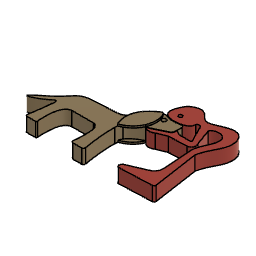
Dog+Human v3 (Autodesk Fusion 360 design; units mm, degrees)
Autodesk Fusion 360 part; units mm, degrees
sketch "Sketch2" plane through (0, 0, 0) normal (0, 0, 1) x (1, 0, 0)
  line L0 (48.3178, -14.7986) -> (66.8883, -14.0451)
  arc A0 (48, -12) -> (47.2858, -13.6689) centre (50.6178, -14.1075) ccw
  line L1 (48, -12) -> (58.7244, -7.4038)
  line L2 (61.7417, -2.4457) -> (60.5774, 13.5743)
  arc A1 (58.7244, -7.4038) -> (61.7417, -2.4457) centre (56.7548, -2.8081) ccw
  line L3 (67.8369, -12.8994) -> (64, 13)
  arc A2 (66.8883, -14.0451) -> (67.8369, -12.8994) centre (66.8477, -13.0459) ccw
  arc A3 (47.2858, -13.6689) -> (48.3178, -14.7986) centre (48.2773, -13.7994) ccw
  spline S0 degree 5 poles (64, 13) (64.0471, 13.236) (64.1458, 13.7046) (64.307, 14.397) (64.5486, 15.2992) (64.8941, 16.3923) (65.2816, 17.4521) (65.7073, 18.4807) (66.1652, 19.4823) (66.6461, 20.4629) (67.1375, 21.4305) (67.6248, 22.3939) (68.0914, 23.3623) (68.5198, 24.344) (68.8918, 25.3461) (69.1895, 26.3733) (69.3965, 27.4267) (69.4986, 28.5028) (69.4851, 29.5927) (69.3499, 30.6803) (69.0922, 31.7424) (68.7145, 32.7515) (68.2224, 33.6784) (67.6229, 34.495) (66.923, 35.1766) (66.1295, 35.7045) (65.2494, 36.0668) (64.2908, 36.2591) (63.2636, 36.2857) (62.18, 36.1608) (61.055, 35.9071) (59.905, 35.5526) (58.7478, 35.1288) (57.6019, 34.6678) (56.4863, 34.1999) (55.4192, 33.7519) (54.4162, 33.3481) (53.4883, 33.0109) (52.6395, 32.7617) (51.8652, 32.6219) (51.15, 32.613) (50.4738, 32.7518) (49.816, 33.047) (49.1613, 33.4942) (48.4996, 34.0735) (47.8215, 34.7497) (47.1154, 35.4716) (46.362, 36.1698) (45.5357, 36.7621) (44.6155, 37.1708) (43.5952, 37.3392) (42.4916, 37.2453) (41.3588, 36.9242) (40.2766, 36.4544) (39.3246, 35.924) (38.5591, 35.4018) (37.9922, 34.91) (37.5608, 34.3854) (37.1497, 33.7029) (36.6699, 32.7597) (36.0857, 31.5062) (35.5413, 30.0769) (35.2161, 28.6525) (35.1938, 27.3301) (35.5233, 26.1827) (36.205, 25.246) (37.2092, 24.5352) (38.4805, 24.0502) (39.9471, 23.7826) (41.5263, 23.7169) (43.1305, 23.8338) (44.6732, 24.1116) (46.0752, 24.5292) (47.2705, 25.0683) (48.2132, 25.7157) (48.8766, 26.4637) (49.1732, 27.1395) (49.262, 27.6892) (49.2618, 28.0748) (49.2469, 28.2723) knots 0 0 0 0 0 0 0.01333333 0.02666667 0.04 0.05333333 0.06666667 0.08 0.09333333 0.10666667 0.12 0.13333333 0.14666667 0.16 0.17333333 0.18666667 0.2 0.21333333 0.22666667 0.24 0.25333333 0.26666667 0.28 0.29333333 0.30666667 0.32 0.33333333 0.34666667 0.36 0.37333333 0.38666667 0.4 0.41333333 0.42666667 0.44 0.45333333 0.46666667 0.48 0.49333333 0.50666667 0.52 0.53333333 0.54666667 0.56 0.57333333 0.58666667 0.6 0.61333333 0.62666667 0.64 0.65333333 0.66666667 0.68 0.69333333 0.70666667 0.72 0.73333333 0.74666667 0.76 0.77333333 0.78666667 0.8 0.81333333 0.82666667 0.84 0.85333333 0.86666667 0.88 0.89333333 0.90666667 0.92 0.93333333 0.94666667 0.96 0.97333333 0.98666667 1 1 1 1 1 1
  arc A4 (51.7725, 28.2723) -> (49.2469, 28.2723) centre (50.5097, 27.6397) ccw
  line L4 (51.7725, 28.2723) -> (56.2933, 19.2488)
  line L5 (55.8463, 18.5249) -> (49.7974, 18.5249)
  arc A5 (55.8463, 18.5249) -> (56.2933, 19.2488) centre (55.8463, 19.0249) ccw
  arc A6 (36.5352, 12.6034) -> (41.8633, 12.6034) centre (39.1992, 15.9969) ccw
  line L6 (36.5352, 12.6034) -> (45.5261, 16.9194)
  arc A7 (45.5261, 16.9194) -> (47.0032, 19.5393) centre (44.3899, 19.2864) ccw
  line L7 (49.2932, 18.6613) -> (47.3781, 19.7793)
  arc A8 (49.2932, 18.6613) -> (49.7974, 18.5249) centre (49.7974, 19.5249) ccw
  arc A9 (47.3781, 19.7793) -> (47.0032, 19.5393) centre (47.2521, 19.5634) ccw
  line L8 (41.8633, 12.6034) -> (47.1907, 14.7614)
  line L9 (47.1907, 14.7614) -> (57.3572, 15.166)
  arc A10 (57.3572, 15.166) -> (59.3412, 19.3874) centre (57.2527, 17.7921) ccw
  line L10 (55.9993, 28.5525) -> (59.3412, 19.3874)
  spline S1 degree 5 poles (55.9993, 28.5525) (56.0014, 28.6403) (56.0224, 28.8148) (56.1046, 29.0731) (56.3157, 29.4108) (56.7472, 29.8172) (57.3391, 30.1944) (58.0744, 30.5148) (58.9263, 30.7421) (59.8582, 30.8379) (60.8246, 30.768) (61.7699, 30.5098) (62.6312, 30.0565) (63.3465, 29.4128) (63.8634, 28.5934) (64.1466, 27.6199) (64.1876, 26.5191) (64.0077, 25.3203) (63.6477, 24.0543) (63.1622, 22.7518) (62.6114, 21.4416) (62.0548, 20.1495) (61.5441, 18.8963) (61.1155, 17.6964) (60.7919, 16.559) (60.5861, 15.4889) (60.5203, 14.6883) (60.5271, 14.1191) (60.5565, 13.7536) (60.5774, 13.5743) knots 0 0 0 0 0 0 0.04 0.08 0.12 0.16 0.2 0.24 0.28 0.32 0.36 0.4 0.44 0.48 0.52 0.56 0.6 0.64 0.68 0.72 0.76 0.8 0.84 0.88 0.92 0.96 1 1 1 1 1 1
  line L11 (36.6253, 12.924) -> (45.4179, 17.1448)
  arc A11 (45.4179, 17.1448) -> (46.7544, 19.5152) centre (44.3899, 19.2864) ccw
  line L12 (46.7544, 19.5152) -> (46.7544, 23)
  spline S2 degree 3 poles (38.1614, 23.9293) (38.1637, 23.9282) (38.166, 23.927) (38.1682, 23.9259) (38.8344, 23.59) (39.8483, 23.4934) (41.1161, 23.5073) (42.4706, 23.5221) (44.0665, 23.6811) (45.4723, 24.0408) knots 0.849842 0.849842 0.849842 0.849842 0.84997 0.84997 0.84997 0.887416 0.887416 0.887416 0.92742 0.92742 0.92742 0.92742
  spline S3 degree 5 poles (38.1614, 23.9293) (38.0904, 23.9626) (37.9463, 24.0275) (37.7243, 24.1199) (37.4165, 24.2331) (37.012, 24.3571) (36.5877, 24.4612) (36.1436, 24.5414) (35.6807, 24.5905) (35.2003, 24.5996) (34.7049, 24.5597) (34.1981, 24.4629) (33.685, 24.3041) (33.1725, 24.083) (32.6687, 23.8027) (32.1817, 23.4686) (31.7196, 23.087) (31.2889, 22.6644) (30.8942, 22.206) (30.5378, 21.7155) (30.2209, 21.1956) (29.999, 20.7573) (29.8502, 20.4163) (29.7589, 20.1836) (29.7151, 20.0659) knots 0 0 0 0 0 0 0.05 0.1 0.15 0.2 0.25 0.3 0.35 0.4 0.45 0.5 0.55 0.6 0.65 0.7 0.75 0.8 0.85 0.9 0.95 1 1 1 1 1 1
  arc A12 (46.7544, 23) -> (45.4723, 24.0408) centre (45.6909, 23) ccw
  line L13 (36.2228, 12.9106) -> (36, 13)
  arc A13 (27.6529, 5.3934) -> (36, 13) centre (23.3259, 18.5248) ccw
  arc A14 (36.2228, 12.9106) -> (36.6253, 12.924) centre (36.4089, 13.3747) ccw
  circle A15 centre (40.6607, 28.1735) radius 1.021
  spline S4 degree 5 poles (27.6042, 3.833) (27.602, 3.6993) (27.5972, 3.3329) (27.594, 2.7215) (27.6001, 1.8426) (27.6274, 0.6635) (27.6817, -0.6876) (27.7608, -2.0969) (27.8648, -3.554) (27.9935, -5.0466) (28.1465, -6.5622) (28.3233, -8.0892) (28.5231, -9.6191) (28.7449, -11.1464) (28.9494, -12.4296) (29.1158, -13.4049) (29.2353, -14.0751) (29.3023, -14.4425) (29.3142, -14.5078) knots 0.094478 0.094478 0.094478 0.094478 0.094478 0.094478 0.133333 0.2 0.266667 0.333333 0.4 0.466667 0.533333 0.6 0.666667 0.733333 0.8 0.866667 0.933333 0.947774 0.947774 0.947774 0.947774 0.947774 0.947774
  spline S5 degree 5 poles (29.7151, 20.0659) (29.7034, 19.9832) (29.6746, 19.8136) (29.6152, 19.5469) (29.5031, 19.166) (29.3072, 18.6479) (29.0541, 18.0893) (28.7433, 17.4946) (28.3758, 16.8732) (27.9541, 16.2381) (27.4813, 15.6035) (26.9607, 14.9833) (26.3957, 14.3898) (25.7897, 13.8308) (25.1457, 13.3105) (24.4663, 12.8304) (23.896, 12.4785) (23.4536, 12.2324) (23.1523, 12.0761) (23, 12) knots 0 0 0 0 0 0 0.066667 0.133333 0.2 0.266667 0.333333 0.4 0.466667 0.533333 0.6 0.666667 0.733333 0.8 0.866667 0.933333 1 1 1 1 1 1
  line L14 (28.3306, -15.688) -> (23.2583, -15.688)
  arc A16 (28.3306, -15.688) -> (29.3142, -14.5078) centre (28.3306, -14.688) ccw
  spline S6 degree 5 poles (22.2762, -14.4996) (22.2937, -14.4079) (22.3426, -14.1433) (22.4165, -13.6959) (22.5039, -13.0476) (22.5884, -12.1739) (22.6483, -11.1641) (22.6776, -10.1178) (22.6815, -9.0523) (22.6668, -7.9917) (22.6403, -6.962) (22.607, -5.9886) (22.5685, -5.0925) (22.5211, -4.2869) (22.4537, -3.5727) (22.3483, -2.9392) (22.1852, -2.3699) (21.9451, -1.8467) (21.6139, -1.3544) (21.2642, -0.9715) (20.9529, -0.691) (20.7213, -0.5052) (20.5955, -0.41) (20.5869, -0.4035) knots 0.073114 0.073114 0.073114 0.073114 0.073114 0.073114 0.1 0.15 0.2 0.25 0.3 0.35 0.4 0.45 0.5 0.55 0.6 0.65 0.7 0.75 0.8 0.85 0.9 0.95 0.953696 0.953696 0.953696 0.953696 0.953696 0.953696
  arc A17 (22.2762, -14.4996) -> (23.2583, -15.688) centre (23.2583, -14.688) ccw
  spline S7 degree 5 poles (23, 12) (22.8644, 11.9727) (22.5949, 11.9202) (22.1952, 11.8479) (21.6715, 11.7643) (21.0295, 11.6804) (20.3913, 11.6155) (19.7391, 11.566) (19.0443, 11.5261) (18.2763, 11.4892) (17.4102, 11.4493) (16.434, 11.4022) (15.3575, 11.3469) (14.2059, 11.2848) (13.0146, 11.2184) (11.822, 11.1509) (10.6644, 11.0845) (9.5691, 11.0198) (8.5482, 10.9547) (7.6011, 10.8845) (6.7187, 10.802) (5.8886, 10.6979) (5.0981, 10.5613) (4.3399, 10.3791) (3.6122, 10.1382) (2.915, 9.8269) (2.2486, 9.4369) (1.6106, 8.9656) (0.9945, 8.4172) (0.3904, 7.8002) (-0.2137, 7.1253) (-0.8314, 6.4042) (-1.4768, 5.6467) (-2.1635, 4.8605) (-2.9029, 4.0519) (-3.7026, 3.2268) (-4.5649, 2.3911) (-5.485, 1.5515) (-6.4493, 0.7165) (-7.4359, -0.1039) (-8.4176, -0.8991) (-9.3652, -1.6583) (-10.2493, -2.3712) (-11.0438, -3.0293) (-11.7284, -3.6258) (-12.2912, -4.1568) (-12.6393, -4.5279) (-12.8423, -4.7758) (-12.9517, -4.9275) (-13, -5) knots 0 0 0 0 0 0 0.022222 0.044444 0.066667 0.088889 0.111111 0.133333 0.155556 0.177778 0.2 0.222222 0.244444 0.266667 0.288889 0.311111 0.333333 0.355556 0.377778 0.4 0.422222 0.444444 0.466667 0.488889 0.511111 0.533333 0.555556 0.577778 0.6 0.622222 0.644444 0.666667 0.688889 0.711111 0.733333 0.755556 0.777778 0.8 0.822222 0.844444 0.866667 0.888889 0.911111 0.933333 0.955556 0.977778 1 1 1 1 1 1
  line L15 (19.3823, 0) -> (7, 0)
  arc A18 (20.5869, -0.4035) -> (19.3823, 0) centre (19.3823, -2) ccw
  spline S8 degree 5 poles (7, 0) (6.9194, -0.0106) (6.7585, -0.036) (6.5184, -0.0869) (6.2009, -0.1804) (5.8085, -0.3411) (5.4216, -0.5488) (5.0422, -0.809) (4.6736, -1.1304) (4.3195, -1.5224) (3.9844, -1.994) (3.6728, -2.5517) (3.389, -3.1985) (3.1369, -3.9332) (2.9197, -4.7508) (2.7395, -5.6427) (2.5971, -6.5958) (2.4917, -7.593) (2.4203, -8.6127) (2.3785, -9.6303) (2.361, -10.62) (2.362, -11.556) (2.3757, -12.4145) (2.3971, -13.1753) (2.422, -13.8233) (2.4482, -14.3503) (2.4691, -14.6725) (2.4846, -14.858) (2.4949, -14.9568) (2.5, -15) knots 0 0 0 0 0 0 0.04 0.08 0.12 0.16 0.2 0.24 0.28 0.32 0.36 0.4 0.44 0.48 0.52 0.56 0.6 0.64 0.68 0.72 0.76 0.8 0.84 0.88 0.92 0.96 1 1 1 1 1 1
  line L16 (2.1088, -15.688) -> (-3, -15.688)
  arc A19 (2.1088, -15.688) -> (2.5, -15) centre (2.1088, -15.2328) ccw
  spline S9 degree 5 poles (-13, -5) (-13.0435, -5.0603) (-13.1155, -5.1721) (-13.1785, -5.313) (-13.1726, -5.4473) (-13.016, -5.5258) (-12.714, -5.5149) (-12.2753, -5.4157) (-11.713, -5.2303) (-11.0438, -4.9629) (-10.2882, -4.6193) (-9.4694, -4.2083) (-8.6131, -3.7416) (-7.7476, -3.2342) (-6.9029, -2.7056) (-6.1081, -2.1769) (-5.3897, -1.6695) (-4.7688, -1.2034) (-4.259, -0.7949) (-3.8636, -0.4553) (-3.5735, -0.1887) (-3.3642, 0.0098) (-3.1943, 0.1557) (-3.0212, 0.2651) (-2.814, 0.3473) (-2.5716, 0.3929) (-2.3181, 0.3778) (-2.088, 0.2729) (-1.9127, 0.0531) (-1.8116, -0.297) (-1.7961, -0.786) (-1.8564, -1.2913) (-1.9431, -1.7347) (-2.0193, -2.0589) (-2.062, -2.2282) knots 0 0 0 0 0 0 0.033333 0.066667 0.1 0.133333 0.166667 0.2 0.233333 0.266667 0.3 0.333333 0.366667 0.4 0.433333 0.466667 0.5 0.533333 0.566667 0.6 0.633333 0.666667 0.7 0.733333 0.766667 0.8 0.833333 0.866667 0.9 0.933333 0.966667 1 1 1 1 1 1
  spline S10 degree 5 poles (-2.062, -2.2282) (-2.0691, -2.3905) (-2.085, -2.7172) (-2.1137, -3.2132) (-2.1621, -3.8867) (-2.2396, -4.749) (-2.3339, -5.6311) (-2.4442, -6.531) (-2.5685, -7.4447) (-2.7031, -8.3651) (-2.843, -9.2835) (-2.9831, -10.1903) (-3.1183, -11.0766) (-3.2443, -11.9348) (-3.3586, -12.7606) (-3.4599, -13.5523) (-3.5303, -14.1582) (-3.5772, -14.5974) (-3.6058, -14.8835) (-3.6194, -15.0248) knots 0 0 0 0 0 0 0.066667 0.133333 0.2 0.266667 0.333333 0.4 0.466667 0.533333 0.6 0.666667 0.733333 0.8 0.866667 0.933333 1 1 1 1 1 1
  arc A20 (-3.6194, -15.0248) -> (-3, -15.688) centre (-3, -15.0671) ccw
  circle A21 centre (38.0321, 21.4887) radius 1.2353
  spline S11 degree 5 poles (28.657, 7.4803) (28.6665, 7.4959) (28.7314, 7.6021) (28.8531, 7.7936) (29.0355, 8.0595) (29.2866, 8.386) (29.6135, 8.755) (29.9756, 9.1162) (30.3812, 9.4834) (30.8349, 9.8666) (31.3354, 10.2687) (31.874, 10.6838) (32.4378, 11.1005) (33.0115, 11.5043) (33.5797, 11.88) (34.1289, 12.2141) (34.6499, 12.4978) (35.1381, 12.7265) (35.5005, 12.8642) (35.7564, 12.942) (35.92, 12.9825) (36, 13) knots 0.191487 0.191487 0.191487 0.191487 0.191487 0.191487 0.2 0.25 0.3 0.35 0.4 0.45 0.5 0.55 0.6 0.65 0.7 0.75 0.8 0.85 0.9 0.95 1 1 1 1 1 1
  arc A22 (28.657, 7.4803) -> (27.6042, 3.833) centre (34.8532, 3.7161) ccw
  spline S12 degree 5 poles (27.6529, 5.3934) (27.5917, 5.5238) (27.4722, 5.787) (27.3016, 6.1893) (27.0915, 6.7405) (26.8583, 7.4542) (26.6562, 8.1925) (26.4881, 8.9545) (26.3586, 9.7387) (26.2744, 10.5428) (26.2431, 11.3628) (26.2709, 12.1929) (26.361, 13.0245) (26.512, 13.8461) (26.7157, 14.6418) (26.9575, 15.3934) (27.2217, 16.0842) (27.495, 16.7037) (27.7703, 17.2505) (28.0523, 17.7383) (28.3566, 18.1947) (28.7027, 18.6509) (29.1081, 19.1349) (29.5815, 19.6613) (30.1188, 20.2273) (30.7077, 20.8181) (31.3311, 21.4121) (31.9707, 21.9853) (32.61, 22.5162) (33.2379, 22.9909) (33.8482, 23.4014) (34.3198, 23.6753) (34.6637, 23.8497) (34.8886, 23.9522) (35, 24) knots 0 0 0 0 0 0 0.033333 0.066667 0.1 0.133333 0.166667 0.2 0.233333 0.266667 0.3 0.333333 0.366667 0.4 0.433333 0.466667 0.5 0.533333 0.566667 0.6 0.633333 0.666667 0.7 0.733333 0.766667 0.8 0.833333 0.866667 0.9 0.933333 0.966667 1 1 1 1 1 1
  spline S13 degree 5 poles (36, 13) (36.0341, 13.0718) (36.1014, 13.2206) (36.1999, 13.4596) (36.3265, 13.8101) (36.4763, 14.3014) (36.6161, 14.8448) (36.7436, 15.4377) (36.8547, 16.0741) (36.9438, 16.7448) (37.0046, 17.4388) (37.0314, 18.1437) (37.0191, 18.8471) (36.9647, 19.5371) (36.8684, 20.2038) (36.7326, 20.8385) (36.5612, 21.4347) (36.3588, 21.9871) (36.13, 22.4919) (35.8784, 22.9471) (35.6062, 23.3521) (35.373, 23.636) (35.1897, 23.8267) (35.0639, 23.9439) (35, 24) knots 0 0 0 0 0 0 0.05 0.1 0.15 0.2 0.25 0.3 0.35 0.4 0.45 0.5 0.55 0.6 0.65 0.7 0.75 0.8 0.85 0.9 0.95 1 1 1 1 1 1
  line L17 (38.6901, 37.6299) -> (33.5795, 25.4813)
  point P0 (65.9185, 18.9318)
  point P1 (68.3564, 23.9877)
  point P2 (69.4704, 29.3006)
  point P3 (67.7566, 34.2708)
  point P4 (64, 36.2418)
  point P5 (57.9019, 34.785)
  point P6 (52.7603, 32.814)
  point P7 (50.1895, 32.8997)
  point P8 (47.3616, 35.2134)
  point P9 (43.1627, 37.2701)
  point P10 (38.3639, 35.2134)
  point P11 (36.1348, 31.5556)
  point P12 (36.8398, 24.8521)
  point P13 (46.4504, 24.7283)
  point P14 (56.8626, 29.8657)
  point P15 (60.5293, 30.7628)
  point P16 (64, 28)
  point P17 (62, 20)
  point P18 (36.4369, 24.4844)
  point P19 (34.1571, 24.4374)
  point P20 (31.5483, 22.9097)
  point P21 (27.6529, 0.1014)
  point P22 (28.2549, -7.4728)
  point P23 (29, 18)
  point P24 (26.74, 14.7614)
  point P25 (22.6616, -10.5608)
  point P26 (22.5451, -4.7345)
  point P27 (22, -2)
  point P28 (20.5071, 11.6302)
  point P29 (17.3179, 11.4444)
  point P30 (10.475, 11.0729)
  point P31 (5.5827, 10.6394)
  point P32 (2.4244, 9.5247)
  point P33 (-0.5171, 6.7689)
  point P34 (-5, 2)
  point P35 (-11, -3)
  point P36 (5.5276, -0.5003)
  point P37 (4, -2)
  point P38 (2.6007, -6.6518)
  point P39 (2.398, -13.1474)
  point P40 (-13, -5.5)
  point P41 (-8.7069, -3.7856)
  point P42 (-3.6194, -0.2295)
  point P43 (-2.9445, 0.2896)
  point P44 (-2.1658, 0.2896)
  point P45 (-2.4514, -6.5629)
  point P46 (-3.1522, -11.313)
  point P47 (29, 8)
  point P48 (30.7092, 9.7573)
  point P49 (33.7462, 11.9769)
  point P50 (26.4858, 9.0233)
  point P51 (26.4476, 13.4549)
  point P52 (27.6529, 17.0078)
  point P53 (29, 19)
  point P54 (32, 22)
  point P55 (36.6856, 15.1825)
  point P56 (37, 19)
  point P57 (36.2228, 22.2741)
  dimension "d1" = 5
  dimension "d2" = 1
  dimension "d3" = 0.5
  dimension "d4" = 1
  dimension "d5" = 0.25
  dimension "d8" = 0.5
  dimension "d11" = 1
  dimension "d12" = 1
  dimension "d13" = 2
  dimension "d14" = 7.25
  constraint tangent L1 A1
  constraint tangent L2 A1
  constraint tangent L0 A2
  constraint tangent L3 A2
  constraint tangent L0 A3
  constraint tangent A0 A3
  constraint equal A2 A3
  constraint tangent A4 L4
  constraint horizontal L5
  constraint tangent L4 A5
  constraint tangent L5 A5
  constraint tangent L6 A7
  constraint tangent L5 A8
  constraint tangent L7 A8
  constraint tangent A7 A9
  constraint tangent L7 A9
  constraint tangent L9 A10
  constraint vertical L12
  constraint tangent L12 A12
  constraint concentric A7 A11
  constraint tangent L11 A11
  constraint tangent L11 A14
  constraint tangent L13 A14
  constraint horizontal L14
  constraint tangent S4 A16
  constraint tangent L14 A16
  constraint tangent L14 A17
  constraint tangent S6 A17
  constraint horizontal L15
  constraint tangent S6 A18
  constraint tangent L15 A18
  constraint parallel L14 L16
  constraint tangent L16 A19
  constraint tangent L16 A20
  constraint tangent S11 A22
  constraint tangent S4 A22
  constraint midpoint P11 L17
  measures "d1" radius of A1
  measures "d2" radius of A2
  measures "d3" radius of A5
  measures "d4" radius of A8
  measures "d5" radius of A9
  measures "d8" radius of A14
  measures "d11" radius of A16
  measures "d12" radius of A17
  measures "d13" radius of A18
  measures "d14" radius of A22
extrude "Extrude1" add sketch "Sketch2" along normal blind 8 contours L0 A0 L1 L2 A1 L3 A2 A3 S0 A4 L4 L5 A5 A6 L6 A7 L7 A8 A9 L8 L9 A10 L10 S1 | L11 A11 L12 S2 S3 A12 L13 A14 S5 S12 S13 | A13 S5 S11 A22 S12 S13 | A13 S4 S5 L14 A16 S6 A17 S7 L15 A18 S8 L16 A19 S9 S10 A20 A22 S12 makes body 1 at (57.9768, -12.0825, 0) makes body 2 at (11.9899, 3.6732, 0)
extrude "Extrude2" add sketch "Sketch2" along normal blind 1 from surface at 8 contours A13 S11 A22 | A13 S5 S11 A22 S12 S13 | S5 S12 bodies 2
extrude "Extrude3" add sketch "Sketch2" along normal blind 1 contours A13 S11 A22 | A13 S5 S11 A22 S12 S13 | S5 S12 bodies 2
